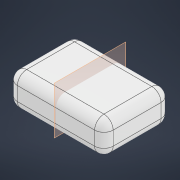
# Autodesk Inventor part: battery
Saved by Autodesk Inventor 2022 (Build 260153000, 153)
## iProperties
Created: 2022-01-31
Part Number: battery
Material: LCP プラスチック
Document SubType Name: Modeling
Designer: shiokaze
Density: 1.626 g/cm^3
Appearance: 滑らか - 白
Mass: 17.7729 g
Surface Area: 29.2667 cm^2
Volume: 10.9305 cm^3
Author: shiokaze
Autodesk Inventor part; units mm, degrees
ref_plane "YZ Plane" through (0, 0, 0) normal (1, 0, 0) x (0, 1, 0)
ref_plane "XZ Plane" through (0, 0, 0) normal (0, 1, 0) x (-1, 0, 0)
ref_plane "XY Plane" through (0, 0, 0) normal (0, 0, 1) x (1, 0, 0)
sketch "スケッチ1" plane through (0, 0, 0) normal (0, 1, 0) x (-1, 0, 0)
  line L0 (15.5, -10.75) -> (-15.5, -10.75)
  line L1 (-15.5, -10.75) -> (-15.5, 10.75)
  line L2 (-15.5, 10.75) -> (15.5, 10.75)
  line L3 (15.5, 10.75) -> (15.5, -10.75)
  line L4 (15.5, -10.75) -> (-15.5, 10.75)
  point P0 (0, 0)
  point P1 (0, 0)
  dimension "d0" = 31
  dimension "d1" = 21.5
  constraints: 10 end point, 2 parallel, 1 coincident, 1 horizontal, 1 midpoint, 1 perpendicular
  measures "d0" distance of L1.end L2.end
  measures "d1" distance of L0.end L1.end
extrude "押し出し1" add sketch "スケッチ1" along normal blind 10.5
fillet "フィレット1" radius 3 11 edges at (15.5, 10.5, 0) (0, 10.5, 10.75) (0, 0, 10.75) (15.5, 5.25, 10.75) (15.5, 0, 0) (15.5, 5.25, -10.75) (0, 10.5, -10.75) (-15.5, 10.5, 0) (-15.5, 5.25, -10.75) (-15.5, 0, 0) (0, 0, -10.75)
ref_plane "作業平面1" through (0, 3, -7.75) normal (1, 0, 0) x (0, 0, -1)
fillet "フィレット2" radius 3 3 edges at (-14.6213, 9.6213, 9.8713) (-14.6213, 0.8787, 9.8713) (-15.5, 5.25, 10.75)
